Autodesk Fusion 360 part; units mm, degrees
(part 2 of 2)
equation "d216 = d200"
equation "d217 = d200"
equation "d218 = d200"
equation "d219 = d200"
equation "d220 = d200"
equation "d237 = tol"
equation "d238 = tol"
equation "d239 = tol"
equation "d240 = tol"
equation "d241 = tol"
equation "d242 = tol"
equation "d243 = tol"
equation "d244 = tol"
equation "d245 = tol"
equation "RCAdia = 9.0 mm"
equation "d265 = RCAdia"
equation "d266 = RCAdia"
equation "d267 = RCAdia"
equation "d269 = d268"
equation "d270 = d268"
named bodies: "PCB", "label"
